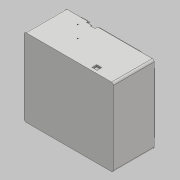
# Autodesk Inventor part: Enclosure
Saved by Autodesk Inventor 2018 (Build 220112000, 112)
## iProperties
Created: 2019-08-08
Part Number: Enclosure
Material: Generic
Document SubType Name: Modeling
Designer: mkivekas
Density: 1 g/cm^3
Appearance: Default
Author: mkivekas
Autodesk Inventor part; units mm, degrees
note: some values were not read from the file. Chosen so that the rebuilt part matches the saved one: direction of "Hole1"; direction of "Hole2".
ref_plane "YZ Plane" through (0, 0, 0) normal (1, 0, 0) x (0, 1, 0)
ref_plane "XZ Plane" through (0, 0, 0) normal (0, 1, 0) x (-1, 0, 0)
ref_plane "XY Plane" through (0, 0, 0) normal (0, 0, 1) x (1, 0, 0)
sketch "Sketch1" plane through (0, 0, 0) normal (0, 1, 0) x (-1, 0, 0)
  line L0 (97, 115.75) -> (-133, 115.75)
  line L1 (-133, 115.75) -> (-133, -84.25)
  line L2 (-133, -84.25) -> (97, -84.25)
  line L3 (97, -84.25) -> (97, 115.75)
  point P0 (0, 0)
  dimension "d0" = 200
  dimension "d1" = 230
  constraints: 8 end point, 2 parallel, 1 horizontal, 1 perpendicular
  measures "d0" distance of L2.end L0.start
  measures "d1" distance of L0.start L0.end
extrude "Extrusion1" add sketch "Sketch1" along normal blind 5
sketch "Sketch2" plane through (0, 5, 0) normal (0, 1, 0) x (1, 0, 0)
  line L0 (-97, -115.75) -> (133, -115.75) projected
  line L1 (133, -115.75) -> (133, 84.25) projected
  line L2 (-97, -115.75) -> (133, -115.75)
  line L3 (133, -115.75) -> (133, 84.25)
  line L4 (133, 84.25) -> (-97, 84.25)
  line L5 (-97, 84.25) -> (-97, -115.75)
  line L6 (-92, -95.75) -> (-92, 64.25)
  line L7 (-92, 64.25) -> (-62, 64.25)
  line L8 (-62, 64.25) -> (-62, 79.25)
  line L9 (-62, 79.25) -> (98, 79.25)
  line L10 (98, 79.25) -> (98, 64.25)
  line L11 (98, 64.25) -> (128, 64.25)
  line L12 (128, 64.25) -> (128, -95.75)
  line L13 (128, -95.75) -> (98, -95.75)
  line L14 (98, -95.75) -> (98, -110.75)
  line L15 (98, -110.75) -> (-62, -110.75)
  line L16 (-62, -110.75) -> (-62, -95.75)
  line L17 (-62, -95.75) -> (-92, -95.75)
  point P0 (0, 0)
  dimension "d4" = 20
  dimension "d5" = 20
  dimension "d6" = 35
  dimension "d7" = 35
  dimension "d8" = 35
  dimension "d9" = 5
  dimension "d10" = 5
  dimension "d11" = 5
  dimension "d12" = 5
  dimension "d13" = 20
  constraints: 32 end point, 8 perpendicular, 4 parallel, 4 point on line, 1 horizontal, 1 vertical
  measures "d4" distance between parallel lines of L2 L17
  measures "d5" distance between parallel lines of L4 L7
  measures "d6" distance between parallel lines of L3 L14
  measures "d7" distance between parallel lines of L3 L10
  measures "d8" distance between parallel lines of L5 L8
  measures "d9" distance between parallel lines of L2 L15
  measures "d10" distance between parallel lines of L5 L6
  measures "d11" distance between parallel lines of L4 L9
  measures "d12" distance between parallel lines of L1 L12
  measures "d13" distance between parallel lines of L2 L13
extrude "Extrusion2" add sketch "Sketch2" along normal blind 100
fillet "Fillet1" radius 5 16 edges at (133, 52.5, -84.25) (-97, 52.5, -84.25) (-97, 52.5, 115.75) (133, 52.5, 115.75) (98, 55, -64.25) (98, 55, -79.25) (128, 55, -64.25) (128, 55, 95.75) (98, 55, 95.75) (98, 55, 110.75) (-62, 55, 95.75) (-62, 55, 110.75) (-92, 55, 95.75) (-92, 55, -64.25) (-62, 55, -64.25) (-62, 55, -79.25)
sketch "Sketch3" plane through (-97, 0, -79.25) normal (-1, 0, 0) x (0, 0, 1)
  line L0 (25, 65) -> (45, 65)
  line L1 (45, 65) -> (45, 53.5)
  line L2 (45, 53.5) -> (25, 53.5)
  line L3 (25, 53.5) -> (25, 65)
  line L4 (65, 65) -> (85, 65)
  line L5 (85, 65) -> (85, 53.5)
  line L6 (85, 53.5) -> (65, 53.5)
  line L7 (65, 53.5) -> (65, 65)
  line L8 (105, 65) -> (121.5, 65)
  line L9 (121.5, 65) -> (121.5, 57.4)
  line L10 (121.5, 57.4) -> (105, 57.4)
  line L11 (105, 57.4) -> (105, 65)
  line L12 (0, 105) -> (190, 105) projected
  line L13 (-5, 105) -> (-5, 0) projected
  line L14 (141.5, 65) -> (158, 65)
  line L15 (158, 65) -> (158, 57.4)
  line L16 (158, 57.4) -> (141.5, 57.4)
  line L17 (141.5, 57.4) -> (141.5, 65)
  line L18 (11.604, 59.25) -> (92.4188, 59.25)
  line L19 (35, 65.5616) -> (35, 51.95)
  circle A0 centre (124.2, 35.2896) radius 2.5
  circle A1 centre (109.6, 35.2896) radius 4.6
  point P0 (79.25, 0)
  point P1 (22.35, 59.25)
  point P2 (47.65, 59.25)
  point P3 (62.35, 59.25)
  point P4 (87.65, 59.25)
  dimension "d17" = 20
  dimension "d18" = 20
  dimension "d19" = 11.5
  dimension "d20" = 11.5
  dimension "d21" = 20
  dimension "d22" = 40
  dimension "d23" = 30
  dimension "d27" = 20
  dimension "d28" = 16.5
  dimension "d29" = 7.6
  dimension "d30" = 0
  dimension "d31" = 16.5
  dimension "d32" = 20
  dimension "d33" = 25.3
  dimension "d34" = 25.3
  dimension "d35" = 25.3
  dimension "d36" = 2.65
  dimension "d48" = 5
  dimension "d73" = 9.2
  constraints: 36 end point, 8 parallel, 6 horizontal, 5 perpendicular, 5 point on line, 2 centre point, 1 vertical
  measures "d17" distance of L0.start L0.end
  measures "d18" distance of L4.start L4.end
  measures "d19" distance of L2.end L0.start
  measures "d20" distance of L6.end L4.start
  measures "d21" distance between parallel lines of L7 L1
  measures "d22" distance between parallel lines of L12 L0
  measures "d23" distance between parallel lines of L13 L3
  measures "d27" distance between parallel lines of L5 L11
  measures "d28" distance of L8.start L8.end
  measures "d29" distance of L8.end L9.end
  measures "d30" distance between parallel lines of L4 L8
  measures "d31" distance of L15.end L16.end
  measures "d32" distance between parallel lines of L17 L9
  measures "d33" distance of point (47.65, 59.25) point (22.35, 59.25)
  measures "d34" distance of point (87.65, 59.25) point (62.35, 59.25)
  measures "d35" diameter of point (22.35, 59.25) L19
  measures "d36" distance from line of L7 point (62.35, 59.25)
  measures "d48" diameter of A0
  measures "d73" diameter of A1
extrude "Extrusion3" cut sketch "Sketch3" against normal blind 100
hole "Hole1" at (-97, 59.25, -56.9) at (-97, 59.25, -31.6) at (-97, 59.25, -16.9) at (-97, 59.25, 8.4) direction (1, 0, 0) diameter 2.459 end up to surface thread size "M3x0.5" class "6H" standard "ISO Metric profile"
sketch "Sketch4" plane through (-92, 0, 115.75) normal (0, 0, 1) x (1, 0, 0)
  line L0 (47.8128, 85) -> (79.3128, 85)
  line L1 (79.3128, 85) -> (79.3128, 53.5)
  line L2 (79.3128, 53.5) -> (47.8128, 53.5)
  line L3 (47.8128, 53.5) -> (47.8128, 85)
  line L4 (0, 105) -> (220, 105) projected
  line L5 (54.3128, 105) -> (79.3128, 105)
  line L6 (79.3128, 105) -> (79.3128, 101)
  line L7 (79.3128, 101) -> (54.3128, 101)
  line L8 (54.3128, 101) -> (54.3128, 105)
  line L9 (79.3128, 101) -> (67.3128, 101)
  line L10 (67.3128, 101) -> (67.3128, 98)
  line L11 (67.3128, 98) -> (79.3128, 98)
  line L12 (79.3128, 98) -> (79.3128, 101)
  line L13 (175.1076, 19.479) -> (162.1076, 19.479)
  line L14 (162.1076, 19.479) -> (162.1076, 7.479)
  line L15 (162.1076, 7.479) -> (175.1076, 7.479)
  line L16 (175.1076, 7.479) -> (175.1076, 19.479)
  line L17 (0, 0) -> (220, 0) projected
  point P0 (92, 0)
  point P1 (79.3128, 103)
  dimension "d50" = 31.5
  dimension "d51" = 31.5
  dimension "d59" = 20
  dimension "d60" = 25
  dimension "d61" = 0
  dimension "d62" = 12
  dimension "d63" = 7
  dimension "d64" = 4
  dimension "d74" = 13
  dimension "d75" = 12
  dimension "d81" = 7.479
  constraints: 32 end point, 8 parallel, 5 horizontal, 4 perpendicular, 2 coincident, 1 midpoint, 1 point on line
  measures "d50" distance of L0.start L0.end
  measures "d51" distance of L0.end L1.end
  measures "d59" distance between parallel lines of L4 L0
  measures "d60" distance of L6.end L7.end
  measures "d61" distance between parallel lines of L6 L1
  measures "d62" distance of L10.end L11.end
  measures "d63" distance between parallel lines of L5 L11
  measures "d64" distance of L7.end L5.start
  measures "d74" distance of L13.start L13.end
  measures "d75" distance of L13.end L14.end
hole "Hole2" at (-44.1872, 85, 115.75) at (-12.6872, 53.5, 115.75) direction (0, 0, -1) diameter 2.621 end up to surface thread size "M3x0.35" class "6H" standard "ISO Metric profile"
extrude "Extrusion4" cut sketch "Sketch4" against normal blind 10 contours L4 L6 L7 L8 | L12 L11 L10 L7 | L16 L15 L14 L13
sketch "Sketch5" plane through (-97, 0, -79.25) normal (-1, 0, 0) x (0, 0, 1)
  line L0 (25, 41.5) -> (33.2, 41.5)
  line L1 (33.2, 41.5) -> (33.2, 38.3)
  line L2 (33.2, 38.3) -> (25, 38.3)
  line L3 (25, 38.3) -> (25, 41.5)
  line L4 (141.5, 57.4) -> (141.5, 65) projected
  line L5 (141.5, 65) -> (158, 65) projected
  line L6 (25, 53.5) -> (25, 65) projected
  line L7 (45, 53.5) -> (25, 53.5) projected
  point P0 (79.25, 0)
  dimension "d67" = 3.2
  dimension "d68" = 8.2
  dimension "d76" = 0
  dimension "d77" = 12
  constraints: 8 end point, 2 parallel, 1 horizontal, 1 perpendicular
  measures "d67" distance of L2.end L0.start
  measures "d68" distance of L0.start L0.end
  measures "d76" distance between parallel lines of L6 L3
  measures "d77" distance between parallel lines of L0 L7
extrude "Extrusion5" cut sketch "Sketch5" against normal blind 10
sketch "Sketch6" plane through (0, 105, 0) normal (0, 1, 0) x (1, 0, 0)
  line L0 (-57, 79.25) -> (93, 79.25) projected
  arc A0 (98, 74.25) -> (93, 79.25) centre (93, 74.25) ccw projected
  line L1 (98, 74.25) -> (98, 69.25) projected
  arc A1 (98, 69.25) -> (103, 64.25) centre (103, 69.25) ccw projected
  line L2 (103, 64.25) -> (123, 64.25) projected
  arc A2 (128, 59.25) -> (123, 64.25) centre (123, 59.25) ccw projected
  line L3 (128, 59.25) -> (128, -90.75) projected
  arc A3 (123, -95.75) -> (128, -90.75) centre (123, -90.75) ccw projected
  line L4 (123, -95.75) -> (103, -95.75) projected
  arc A4 (103, -95.75) -> (98, -100.75) centre (103, -100.75) ccw projected
  arc A5 (93, -110.75) -> (98, -105.75) centre (93, -105.75) ccw projected
  line L5 (98, -100.75) -> (98, -105.75) projected
  line L6 (93, -110.75) -> (-12.6872, -110.75) projected
  line L7 (-37.6872, -110.75) -> (-57, -110.75) projected
  arc A6 (-62, -105.75) -> (-57, -110.75) centre (-57, -105.75) ccw projected
  line L8 (-62, -105.75) -> (-62, -100.75) projected
  arc A7 (-62, -100.75) -> (-67, -95.75) centre (-67, -100.75) ccw projected
  line L9 (-67, -95.75) -> (-87, -95.75) projected
  arc A8 (-92, -90.75) -> (-87, -95.75) centre (-87, -90.75) ccw projected
  line L10 (-92, -90.75) -> (-92, 59.25) projected
  arc A9 (-87, 64.25) -> (-92, 59.25) centre (-87, 59.25) ccw projected
  line L11 (-87, 64.25) -> (-67, 64.25) projected
  arc A10 (-67, 64.25) -> (-62, 69.25) centre (-67, 69.25) ccw projected
  line L12 (-62, 69.25) -> (-62, 74.25) projected
  arc A11 (-57, 79.25) -> (-62, 74.25) centre (-57, 74.25) ccw projected
  line L13 (-12.6872, -112.75) -> (93, -112.75)
  arc A12 (93, -112.75) -> (100, -105.75) centre (93, -105.75) ccw
  line L14 (100, -105.75) -> (100, -100.75)
  arc A13 (103, -97.75) -> (100, -100.75) centre (103, -100.75) ccw
  line L15 (103, -97.75) -> (123, -97.75)
  arc A14 (123, -97.75) -> (130, -90.75) centre (123, -90.75) ccw
  line L16 (130, -90.75) -> (130, 59.25)
  arc A15 (130, 59.25) -> (123, 66.25) centre (123, 59.25) ccw
  line L17 (123, 66.25) -> (103, 66.25)
  arc A16 (100, 69.25) -> (103, 66.25) centre (103, 69.25) ccw
  line L18 (100, 69.25) -> (100, 74.25)
  arc A17 (100, 74.25) -> (93, 81.25) centre (93, 74.25) ccw
  line L19 (93, 81.25) -> (-57, 81.25)
  arc A18 (-57, 81.25) -> (-64, 74.25) centre (-57, 74.25) ccw
  line L20 (-64, 74.25) -> (-64, 69.25)
  arc A19 (-67, 66.25) -> (-64, 69.25) centre (-67, 69.25) ccw
  line L21 (-67, 66.25) -> (-87, 66.25)
  arc A20 (-87, 66.25) -> (-94, 59.25) centre (-87, 59.25) ccw
  line L22 (-94, 59.25) -> (-94, -90.75)
  arc A21 (-94, -90.75) -> (-87, -97.75) centre (-87, -90.75) ccw
  line L23 (-87, -97.75) -> (-67, -97.75)
  arc A22 (-64, -100.75) -> (-67, -97.75) centre (-67, -100.75) ccw
  line L24 (-64, -100.75) -> (-64, -105.75)
  arc A23 (-64, -105.75) -> (-57, -112.75) centre (-57, -105.75) ccw
  line L25 (-57, -112.75) -> (-37.6872, -112.75)
  line L26 (-37.6872, -115.75) -> (-37.6872, -110.75) projected
  line L27 (-37.6872, -112.75) -> (-37.6872, -110.75)
  line L28 (-12.6872, -110.75) -> (-12.6872, -115.75) projected
  line L29 (-12.6872, -112.75) -> (-12.6872, -110.75)
  point P0 (0, 0)
  dimension "d78" = 2
  constraints: 30 end point, 24 point on circle, 12 centre point, 2 collinear, 24 other
  measures "d78" distance between parallel lines of L0 L19
extrude "Extrusion6" add sketch "Sketch6" along normal blind 4
body "Solid1"
